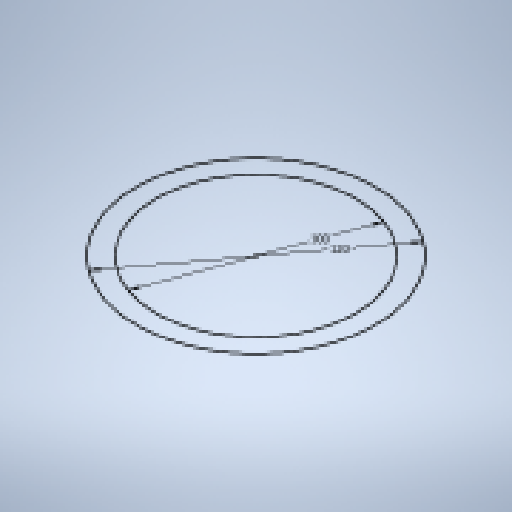
# Autodesk Inventor part: Bottom_Stand
Saved by Autodesk Inventor 2025.1 (Build 291241000, 241)
## iProperties
Created: 2026-04-16
Part Number: Bottom_Stand
Material: Generic
Document SubType Name: Modeling
Designer: ryand
Density: 1 g/cm^3
Appearance: Default
Author: ryand
Autodesk Inventor part; units mm, degrees
ref_plane "YZ Plane" through (0, 0, 0) normal (1, 0, 0) x (0, 1, 0)
ref_plane "XZ Plane" through (0, 0, 0) normal (0, 1, 0) x (-1, 0, 0)
ref_plane "XY Plane" through (0, 0, 0) normal (0, 0, 1) x (1, 0, 0)
sketch "Sketch1" plane through (0, 0, 0) normal (0, 1, 0) x (-1, 0, 0)
  circle A0 centre (0, 0) radius 60
  circle A1 centre (0, 0) radius 50
  circle A2 centre (0, 0) radius 5
  line L0 (5, 0) -> (-5, 0)
  line L1 (-5, 0) -> (-5, -50)
  line L2 (-5, -50) -> (5, -50)
  line L3 (5, -50) -> (5, 0)
  line L4 (2.5, -4.3301) -> (45.8013, 20.6699)
  line L5 (40.8013, 29.3301) -> (-2.5, 4.3301)
  line L6 (2.5, 4.3301) -> (-40.8013, 29.3301)
  line L7 (-45.8013, 20.6699) -> (-2.5, -4.3301)
  point P0 (0, 5.7735)
  point P1 (-40.5842, 29.2048)
  point P2 (40.5842, 29.2048)
  point P3 (5, -2.8868)
  point P4 (45.5842, 20.5446)
  point P5 (5, -49.7494)
  point P6 (-5, -2.8868)
  point P7 (-5, -49.7494)
  point P8 (-45.5842, 20.5446)
  dimension "d2" = 10
  dimension "d0" = 120
  dimension "d1" = 100
  dimension "d3" = 50
  dimension "d6" = 360
  constraints: 16 end point, 3 coincident, 2 centre point, 2 parallel, 1 horizontal, 1 horizontal alignment, 1 perpendicular, 21 other
  measures "d0" diameter of A0
  measures "d1" diameter of A1
  measures "d3" distance of L1.end L0.end
extrude "Extrusion1" add sketch "Sketch1" along normal blind 5 contours A0 | L4 L3 A2 L6 L5 A1 | L3 L2 A1 | A1 L1 L7 A2 L4 L3 | L4 A2 L3 | L2 L1 A1 | L6 L5 A2 L1 L7 A1 | L6 A2 L5 | L0 A2 | A2 L0 | A2 L7 L1
sketch "Sketch3" plane through (0, 0, 0) normal (0, -1, 0) x (1, 0, 0)
  circle A0 centre (0, -70) radius 1.75
  arc A1 (-5, -70) -> (5, -70) centre (0, -70) ccw
  line L0 (-5, -70) -> (-5, -59.7913)
  circle A2 centre (0, 0) radius 60 projected
  line L1 (-5, -70) -> (5.2087, -70) construction
  line L2 (5, -70) -> (5, -59.7913)
  arc A3 (-5, -59.7913) -> (5, -59.7913) centre (0, 0) ccw
  circle A4 centre (60.6218, 35) radius 1.75
  line L3 (63.1218, 30.6699) -> (58.0174, 39.5109) construction
  arc A5 (63.1218, 30.6699) -> (58.1218, 39.3301) centre (60.6218, 35) ccw
  line L4 (58.1218, 39.3301) -> (49.2808, 34.2258)
  line L5 (63.1218, 30.6699) -> (54.2808, 25.5655)
  arc A6 (54.2808, 25.5655) -> (49.2808, 34.2258) centre (0, 0) ccw
  circle A7 centre (-60.6218, 35) radius 1.75
  line L6 (-58.1218, 39.3301) -> (-63.2261, 30.4891) construction
  arc A8 (-58.1218, 39.3301) -> (-63.1218, 30.6699) centre (-60.6218, 35) ccw
  line L7 (-63.1218, 30.6699) -> (-54.2808, 25.5655)
  line L8 (-58.1218, 39.3301) -> (-49.2808, 34.2258)
  arc A9 (-49.2808, 34.2258) -> (-54.2808, 25.5655) centre (0, 0) ccw
  dimension "d10" = 3.5
  dimension "d12" = 5
  dimension "d21" = 90
  dimension "d24" = 360
  constraints: 18 end point, 14 point on circle, 9 centre point, 4 coincident, 1 horizontal, 1 perpendicular, 43 other
  measures "d10" diameter of A0
  measures "d12" distance of L2.start A0.centre
  measures "d21" angle of L1 L0
extrude "Extrusion3" add sketch "Sketch3" against normal blind 35 contours L0 A2 L2 A1 | L7 A8 L8 A2 | A2 L4 A5 L5
sketch "Sketch4" plane through (58.1218, 0, 39.3301) normal (-0.5, 0, 0.8660254) x (0.8660254, 0, 0.5)
  line L0 (0, 0) -> (0, 35) projected
  line L1 (-10.2087, 5) -> (-10.2087, 35) projected
  line L2 (-10.2087, 5) -> (-95.5655, 5) projected
  line L3 (-10.2087, 35) -> (0, 35) projected
  line L4 (-8.4587, 32.5) -> (-3.4587, 32.5)
  line L5 (-3.4587, 32.5) -> (-3.4587, 7.5)
  line L6 (-3.4587, 7.5) -> (-8.4587, 7.5)
  line L7 (-8.4587, 7.5) -> (-8.4587, 32.5)
  line L8 (-8.4587, 7.5) -> (-1.3876, 7.5) construction
  line L9 (-8.4587, 7.5) -> (-3.4587, 16.1603)
  line L10 (-8.4587, 7.5) -> (1.5413, 7.5) construction
  line L11 (-3.4587, 16.1603) -> (-8.4587, 24.8205)
  line L12 (-8.4587, 24.8205) -> (-3.4587, 32.5)
  line L13 (-3.4587, 32.5) -> (-2.6207, 31.9544)
  line L14 (-2.6207, 31.9544) -> (-4.2967, 33.0456)
  line L15 (-4.2967, 33.0456) -> (-8.4587, 26.6533)
  line L16 (-8.4587, 24.8205) -> (-7.6207, 24.2749)
  line L17 (-7.2859, 24.7891) -> (-2.6207, 31.9544)
  line L18 (-3.4587, 16.1603) -> (-2.5927, 16.6603)
  line L19 (-3.4587, 16.1603) -> (-2.4587, 16.1603) construction
  line L20 (-2.5927, 16.6603) -> (-4.3247, 15.6603)
  line L21 (-4.3247, 15.6603) -> (-8.4587, 22.8205)
  line L22 (-7.2859, 24.7891) -> (-2.5927, 16.6603)
  line L23 (-8.4587, 7.5) -> (-9.3247, 8)
  line L24 (-9.3247, 8) -> (-7.5927, 7)
  line L25 (-7.5927, 7) -> (-2.5927, 15.6603)
  line L26 (-2.5927, 15.6603) -> (-4.3247, 16.6603)
  line L27 (-4.3247, 16.6603) -> (-9.3247, 8)
  line L28 (-9.3247, 8) -> (-7.3247, 8) construction
  point P0 (-70, 0)
  dimension "d28" = 10.2087
  dimension "d29" = 30
  dimension "d30" = 5
  dimension "d31" = 25
  dimension "d32" = 2.5
  dimension "d33" = 1.75
  dimension "d37" = 60
  dimension "d38" = 120
  dimension "d40" = 1
  dimension "d41" = 2
  dimension "d45" = 1
  dimension "d46" = 30
  dimension "d47" = 2
  dimension "d48" = 1
  dimension "d49" = 2
  dimension "d50" = 30
  constraints: 50 end point, 7 parallel, 6 perpendicular, 5 horizontal, 5 point on line, 3 equal length, 1 collinear
  measures "d28" distance between parallel lines of L0 L1
  measures "d29" distance between parallel lines of L2 L3
  measures "d30" distance of L5.end L6.end
  measures "d31" distance of L4.end L5.end
  measures "d32" distance between parallel lines of L3 L4
  measures "d33" distance between parallel lines of L1 L7
  measures "d37" angle of L10 L9
  measures "d38" angle of L11 L9
  measures "d40" distance of L4.end L13.end
  measures "d41" distance of L13.end L14.end
  measures "d45" distance of L9.end L18.end
  measures "d46" angle of L19 L18
  measures "d47" distance of L18.end L20.end
  measures "d48" distance of L6.end L23.end
  measures "d49" distance of L24.start L24.end
  measures "d50" angle of L24 L28
extrude "Extrusion4" cut sketch "Sketch4" against normal blind 10 contours L4 L15 L7 | L4 L12 L7 L15 | L5 L17 L22 L11 L12 | L11 L26 L27 L21 L7 | L5 L22 L17 | L21 L27 L7 | L5 L25 L6 L9 | L9 L7 L27 L21 L20 | L20 L21 L27 L26 | L5 L6 L25
body "Solid1"
